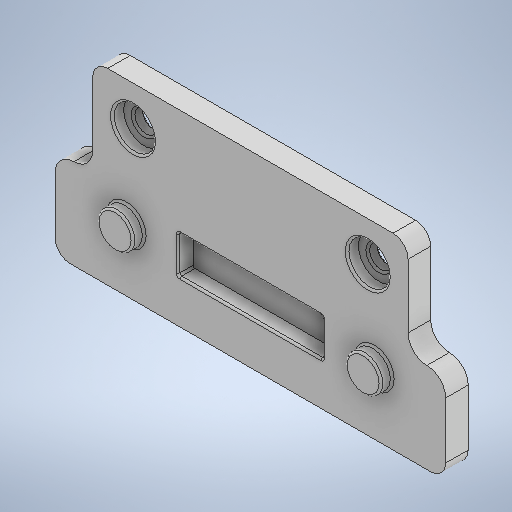
# Autodesk Inventor part: 5RM_belt_clip
Saved by Autodesk Inventor 2025 (Build 290162010, 162A)
## iProperties
Created: 2025-11-18
Part Number: 5RM_belt_clip
Material: Generic
Document SubType Name: Modeling
Designer: vaugerbird
Density: 1 g/cm^3
Appearance: Default
Author: vaugerbird
Autodesk Inventor part; units mm, degrees
ref_plane "YZ Plane" through (0, 0, 0) normal (1, 0, 0) x (0, 1, 0)
ref_plane "XZ Plane" through (0, 0, 0) normal (0, 1, 0) x (-1, 0, 0)
ref_plane "XY Plane" through (0, 0, 0) normal (0, 0, 1) x (1, 0, 0)
sketch "Sketch1" plane through (0, 0, 0) normal (0, 0, 1) x (1, 0, 0)
  line L0 (2, 0) -> (50, 0)
  line L1 (52, 2) -> (52, 9.5)
  line L2 (49.5, 12) -> (49.5, 12)
  line L3 (0, 9.5) -> (0, 2)
  line L4 (2.5, 12) -> (2.5, 12)
  line L5 (52, 12) -> (47, 12)
  line L6 (47, 14.5) -> (47, 23)
  line L7 (45, 25) -> (7, 25)
  line L8 (5, 23) -> (5, 14.5)
  arc A0 (7, 25) -> (5, 23) centre (7, 23) ccw
  arc A1 (47, 23) -> (45, 25) centre (45, 23) ccw
  arc A2 (0, 2) -> (2, 0) centre (2, 2) ccw
  arc A3 (50, 0) -> (52, 2) centre (50, 2) ccw
  arc A4 (2.5, 12) -> (5, 14.5) centre (2.5, 14.5) ccw
  arc A5 (2.5, 12) -> (0, 9.5) centre (2.5, 9.5) ccw
  arc A6 (47, 14.5) -> (49.5, 12) centre (49.5, 14.5) ccw
  arc A7 (52, 9.5) -> (49.5, 12) centre (49.5, 9.5) ccw
  point P0 (0, 0)
  point P1 (52, 0)
  point P2 (0, 12)
  point P3 (5, 12)
  point P4 (47, 25)
  point P5 (5, 25)
  dimension "d6" = 52
  dimension "d7" = 12
  dimension "d8" = 5
  dimension "d9" = 5
  dimension "d10" = 13
  dimension "d11" = 42
  dimension "d12" = 2
  dimension "d13" = 2
  dimension "d14" = 2.5
  constraints: 18 end point, 18 point on line, 16 point on circle, 16 tangent, 8 centre point, 5 equal radius, 4 perpendicular, 1 horizontal, 1 vertical
  measures "d6" distance of point (0, 0) point (52, 0)
  measures "d7" distance of point (52, 0) L5.start
  measures "d8" distance of point (0, 12) point (5, 12)
  measures "d9" distance of L5.start L5.end
  measures "d10" distance of L5.end point (47, 25)
  measures "d11" distance of point (47, 25) point (5, 25)
  measures "d12" radius of A0
  measures "d13" radius of A2
  measures "d14" radius of A4
extrude "Extrusion1" add sketch "Sketch1" along normal blind 3
sketch "Sketch2" plane through (0, 0, 3) normal (0, 0, 1) x (1, 0, 0)
  line L0 (0, 0) -> (0, 12)
  line L1 (52, 12) -> (52, 0)
  line L2 (52, 0) -> (0, 0)
  line L3 (0, 0) -> (0.25, 0)
  line L4 (52, 0) -> (51.75, 0)
  line L5 (0.25, 0) -> (51.75, 0)
  circle A0 centre (9.49, 8.25) radius 2.375
  circle A1 centre (42.51, 8.25) radius 2.375
  line L6 (0, 12) -> (52, 12)
  line L7 (2, 0) -> (50, 0) projected
  line L8 (0, 0) -> (2, 0)
  arc A2 (50, 0) -> (52, 2) centre (50, 2) ccw projected
  line L9 (50, 0) -> (52, 0)
  arc A3 (2.5, 12) -> (0, 9.5) centre (2.5, 9.5) ccw projected
  line L10 (2.5, 12) -> (0, 12)
  arc A4 (47, 14.5) -> (49.5, 12) centre (49.5, 14.5) ccw projected
  line L11 (52, 12) -> (49.5, 12)
  line L12 (9.49, 12) -> (9.49, 8.25)
  line L13 (0, 9.5) -> (0, 12)
  arc A5 (52, 9.5) -> (49.5, 12) centre (49.5, 9.5) ccw projected
  line L14 (52, 9.5) -> (52, 12)
  line L15 (52, 12) -> (42.51, 12)
  line L16 (42.51, 12) -> (42.51, 8.25)
  line L17 (0, 12) -> (9.49, 12)
  dimension "d17" = 12
  dimension "d18" = 52
  dimension "d22" = 3.75
  dimension "d23" = 4.75
  dimension "d24" = 9.49
  dimension "d25" = 9.49
  dimension "d26" = 3.75
  dimension "d27" = 4.75
  constraints: 34 end point, 4 collinear, 3 vertical, 2 centre point, 2 coincident, 2 perpendicular, 2 point on line, 2 tangent, 1 horizontal
  measures "d17" distance of L1.start L1.end
  measures "d18" distance of L0.end L1.start
  measures "d22" distance of L16.end L15.end
  measures "d23" diameter of A1
  measures "d24" distance of L1.start L15.end
  measures "d25" distance of L0.end L12.start
  measures "d26" distance of L12.start L12.end
  measures "d27" diameter of A0
extrude "Extrusion2" add sketch "Sketch2" along normal blind 1.5 contours A1 | A0
sketch "Sketch3" plane through (0, 0, 3) normal (0, 0, 1) x (1, 0, 0)
  arc A0 (52, 9.5) -> (49.5, 12) centre (49.5, 9.5) ccw projected
  line L0 (52, 9.5) -> (52, 12)
  line L1 (52, 12) -> (0, 12)
  arc A1 (2.5, 12) -> (0, 9.5) centre (2.5, 9.5) ccw projected
  line L2 (0, 12) -> (0, 9.5)
  arc A2 (2.5, 12) -> (5, 14.5) centre (2.5, 14.5) ccw projected
  line L3 (2.5, 12) -> (2.5, 19.75)
  line L4 (2.5, 19.75) -> (49.5, 19.75)
  line L5 (49.5, 19.75) -> (49.5, 12)
  line L6 (26, 19.75) -> (41.625, 19.75)
  line L7 (26, 19.75) -> (10.375, 19.75)
  circle A3 centre (10.375, 19.75) radius 1.5
  circle A4 centre (41.625, 19.75) radius 1.5
  circle A5 centre (10.375, 19.75) radius 2.75
  circle A6 centre (41.625, 19.75) radius 2.75
  point P0 (0, 0)
  dimension "d30" = 2.5
  dimension "d31" = 7.75
  dimension "d32" = 47
  dimension "d33" = 15.625
  dimension "d34" = 15.625
  dimension "d35" = 3
  dimension "d36" = 3
  dimension "d37" = 5.5
  dimension "d38" = 5.5
  constraints: 16 end point, 4 centre point, 4 coincident, 3 point on line, 3 vertical, 2 perpendicular, 2 tangent, 1 midpoint, 1 point on circle
  measures "d30" distance of L1.end L2.end
  measures "d31" distance of L3.start L3.end
  measures "d32" distance of L3.end L4.end
  measures "d33" distance of L6.start L6.end
  measures "d34" distance of L6.start L7.end
  measures "d35" diameter of A3
  measures "d36" diameter of A4
  measures "d37" diameter of A5
  measures "d38" diameter of A6
extrude "Extrusion3" cut sketch "Sketch3" against normal up to surface (3 mm away) contours A4 L4 | L4 A4 | A3 L4 | L4 A3
extrude "Extrusion4" cut sketch "Sketch3" against normal blind 1.5 contours A6 L4 A4 | L4 A4 A6 | A5 L4 A3 | L4 A3 A5
sketch "Sketch4" plane through (0, 0, 3) normal (0, 0, 1) x (1, 0, 0)
  circle A0 centre (9.49, 8.25) radius 2.2 projected
  circle A1 centre (42.51, 8.25) radius 2.2 projected
  line L0 (16.375, 8.25) -> (16.375, 10.5)
  line L1 (16.375, 8.25) -> (16.375, 6)
  line L2 (16.625, 5.75) -> (35.375, 5.75)
  line L3 (35.625, 6) -> (35.625, 10.5)
  line L4 (35.375, 10.75) -> (16.625, 10.75)
  arc A2 (16.625, 10.75) -> (16.375, 10.5) centre (16.625, 10.5) ccw
  arc A3 (16.375, 6) -> (16.625, 5.75) centre (16.625, 6) ccw
  arc A4 (35.375, 5.75) -> (35.625, 6) centre (35.375, 6) ccw
  arc A5 (35.625, 10.5) -> (35.375, 10.75) centre (35.375, 10.5) ccw
  line L5 (9.49, 8.25) -> (42.51, 8.25)
  line L6 (26, 8.25) -> (16.375, 8.25)
  line L7 (26, 8.25) -> (26, 10.75)
  point P0 (0, 0)
  point P1 (16.375, 10.75)
  point P2 (16.375, 5.75)
  dimension "d48" = 2.5
  dimension "d49" = 2.5
  dimension "d50" = 0.25
  dimension "d53" = 2.5
  dimension "d55" = 18.75
  constraints: 16 end point, 8 point on circle, 8 tangent, 4 centre point, 4 point on line, 3 equal radius, 3 perpendicular, 2 midpoint, 2 vertical, 1 collinear, 1 horizontal
  measures "d48" distance of L0.start point (16.375, 10.75)
  measures "d49" distance of L0.start point (16.375, 5.75)
  measures "d50" radius of A2
  measures "d53" distance of L6.start L7.end
  measures "d55" distance of L4.start L4.end
extrude "Extrusion5" cut sketch "Sketch4" against normal blind 2 contours L0 A2 L4 L7 L5 | L5 L3 A4 L2 A3 L1 | L7 L4 A5 L3 L5
fillet "Fillet3" radius 0.25 18 edges at (7.115, 8.25, 4.5) (7.115, 8.25, 3) (16.375, 8.25, 3) (26, 10.75, 3) (16.4482, 10.6768, 3) (16.4482, 5.8232, 3) (26, 5.75, 3) (35.5518, 5.8232, 3) (35.625, 8.25, 3) (35.5518, 10.6768, 3) (40.135, 8.25, 4.5) (40.135, 8.25, 3) (38.875, 19.75, 3) (40.125, 19.75, 1.5) (7.625, 19.75, 3) (8.875, 19.75, 1.5) (40.125, 19.75, 0) (8.875, 19.75, 0)
body "Solid1"
